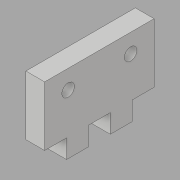
# Autodesk Inventor part: g_mount 1
Saved by Autodesk Inventor 2019 (Build 230136000, 136)
## iProperties
Created: 2021-11-01
Part Number: g_mount 1
Material: Generic
Document SubType Name: Modeling
Designer: Mohamed
Density: 1 g/cm^3
Appearance: Default
Author: Mohamed
Autodesk Inventor part; units mm, degrees
ref_plane "YZ Plane" through (0, 0, 0) normal (1, 0, 0) x (0, 1, 0)
ref_plane "XZ Plane" through (0, 0, 0) normal (0, 1, 0) x (-1, 0, 0)
ref_plane "XY Plane" through (0, 0, 0) normal (0, 0, 1) x (1, 0, 0)
sketch "Sketch1" plane through (0, 0, 0) normal (1, 0, 0) x (0, 1, 0)
  line L0 (0, 0) -> (25, 0)
  line L1 (25, 0) -> (25, -35)
  line L2 (25, -35) -> (0, -35)
  line L3 (0, -35) -> (0, 0)
  circle A0 centre (19, -7.5) radius 2
  circle A1 centre (19, -27.5) radius 2
  dimension "d0" = 25
  dimension "d1" = 35
  dimension "d5" = 4
  dimension "d6" = 4
  constraints: 8 end point, 2 centre point, 2 parallel, 1 horizontal, 1 perpendicular
  measures "d0" distance of L1.end L2.end
  measures "d1" distance of L0.end L1.end
  measures "d5" diameter of A0
  measures "d6" diameter of A1
extrude "Extrusion1" add sketch "Sketch1" along normal blind 6
sketch "Sketch2" plane through (6, 0, 0) normal (1, 0, 0) x (0, 0, -1)
  line L0 (0, 0) -> (7, 0)
  line L1 (7, 0) -> (7, 6)
  line L2 (7, 6) -> (0, 6)
  line L3 (0, 6) -> (0, 0)
  dimension "d9" = 7
  dimension "d10" = 6
  constraints: 8 end point, 2 parallel, 1 horizontal, 1 perpendicular
  measures "d9" distance of L2.end L1.end
  measures "d10" distance of L1.end L0.end
extrude "Extrusion2" cut sketch "Sketch2" against normal blind 6
pattern_linear "Rectangular Pattern1" count 3 spacing 14 along (0, 0, -1) of "Extrusion2"
body "Solid1"
